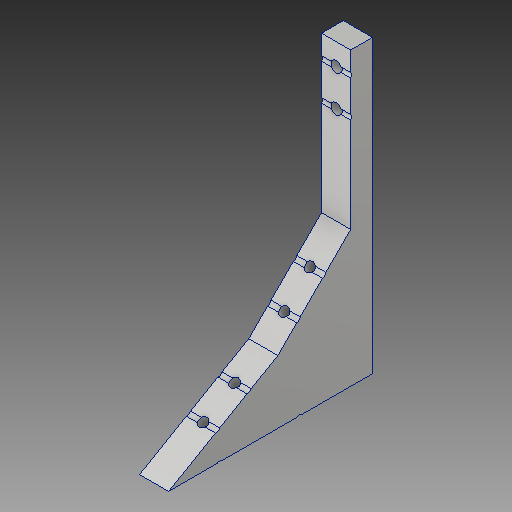
# Autodesk Inventor part: 앞판센서막이
Saved by Autodesk Inventor 2017 (Build 210142000, 142)
## iProperties
Part Number: 앞판센서막이
Material: 알루미늄 6061
Document SubType Name: Modeling
Designer: minom
Density: 2.7 g/cm^3
Appearance: 알루미늄 - 평지
Mass: 18.1843 g
Surface Area: 55.7658 cm^2
Volume: 6.73492 cm^3
Author: minom
Autodesk Inventor part; units mm, degrees
ref_plane "YZ Plane" through (0, 0, 0) normal (1, 0, 0) x (0, 1, 0)
ref_plane "XZ Plane" through (0, 0, 0) normal (0, 1, 0) x (-1, 0, 0)
sketch "스케치1" plane through (0, 0, 0) normal (1, 0, 0) x (0, 1, 0)
  line L0 (0, 0) -> (0, -30)
  line L1 (0, -30) -> (0, -50)
  line L2 (0, -50) -> (37.3205, -50)
  line L3 (0, 0) -> (17.3205, -30)
  line L4 (0, 0) -> (34.641, 0) construction
  line L5 (17.3205, -30) -> (37.3205, -50)
  line L6 (17.3205, -30) -> (43.1906, -30) construction
  line L7 (0, -30) -> (17.3205, -30)
  dimension "d0" = 30
  dimension "d1" = 20
  dimension "d2" = 60
  dimension "d3" = 45
  constraints: 16 end point, 2 horizontal, 1 collinear, 1 equal length, 1 perpendicular, 1 point on line, 1 vertical
  measures "d0" distance of L0.start L0.end
  measures "d1" distance of L0.end L1.end
  measures "d2" angle of L3 L4
  measures "d3" angle of L5 L6
extrude "돌출2" add sketch "스케치1" along normal blind 8
sketch "스케치7" plane through (8, 0, 0) normal (1, 0, 0) x (0, 0, -1)
  line L0 (50, 0) -> (50, 37.3205) projected
  line L1 (50, 0) -> (56, 0)
  line L2 (56, 0) -> (56, 80)
  line L3 (56, 80) -> (50, 80)
  line L4 (50, 80) -> (50, 0)
  point P0 (0, 0)
  dimension "d47" = 6
  dimension "d48" = 80
  constraints: 8 end point, 2 parallel, 1 horizontal, 1 perpendicular
  measures "d47" distance of L3.end L2.end
  measures "d48" distance of L2.end L1.end
extrude "돌출9" add sketch "스케치7" against normal blind 8
sketch "스케치2" plane through (0, 0, -50) normal (0, -1, 0) x (1, 0, 0)
  line L0 (0, 50) -> (0, -6) projected
  line L1 (8, 50) -> (8, -6) projected
  line L2 (0, 50) -> (8, 50) projected
  circle A0 centre (4, 36) radius 1.25
  circle A1 centre (4, 14) radius 1.25
  line L3 (8, -6) -> (0, -6) projected
  dimension "d9" = 2.5
  dimension "d10" = 2.5
  dimension "d11" = 14
  dimension "d12" = 4
  dimension "d14" = 4
  constraints: 2 centre point
  measures "d9" diameter of A0
  measures "d10" diameter of A1
  measures "d11" distance from line of L2 A0.centre
  measures "d12" distance from line of L1 A0.centre
  measures "d14" distance from line of A1.centre L1
extrude "돌출3" cut sketch "스케치2" against normal blind 4.1 contours A0 | A1
sketch "스케치3" plane through (0, 0, 0) normal (-1, 0, 0) x (0, 0, 1)
  line L0 (0, 0) -> (-56, 0) projected
  line L1 (-30, 17.3205) -> (0, 0) projected
  line L2 (-50, 37.3205) -> (-30, 17.3205) projected
  line L3 (-32.4561, 14.1197) -> (-14.9282, 4)
  line L4 (-14.9282, 4) -> (-52, 4)
  line L5 (-52, 4) -> (-52, 33.6637)
  line L6 (-52, 33.6637) -> (-32.4561, 14.1197)
  line L7 (-50, 37.3205) -> (-50, 80) projected
  line L8 (-50, 80) -> (-56, 80) projected
  line L9 (-56, 80) -> (-56, 0) projected
  dimension "d17" = 4
  dimension "d51" = 4
  dimension "d60" = 4
  constraints: 8 end point, 1 other
  measures "d17" distance between parallel lines of L2 L6
  measures "d51" distance between parallel lines of L5 L9
  measures "d60" distance between parallel lines of L1 L3
extrude "돌출4" cut sketch "스케치3" against normal blind 7 contours L3 L4 L5 L6
sketch "스케치5" plane through (0, 17.3205, -30) normal (0, 0.7071068, 0.7071068) x (1, 0, 0)
  circle A0 centre (4, 8) radius 1.6 projected
  circle A1 centre (-36, 18) radius 1.6 projected
  circle A2 centre (-255.8, 18) radius 1.6 projected
  circle A3 centre (-295.8, 18) radius 1.6 projected
  circle A4 centre (-295.8, 8) radius 1.6 projected
  circle A5 centre (-255.8, 8) radius 1.6 projected
  circle A6 centre (-36, 8) radius 1.6 projected
  circle A7 centre (4, 18) radius 1.6 projected
  line L0 (-300.9, 27) -> (9.1, 27) projected
  line L1 (-300.9, 1) -> (-300.9, 27) projected
  line L2 (9.1, 1) -> (-137.9, 1) projected
  line L3 (-153.9, 1) -> (-300.9, 1) projected
  line L4 (9.1, 27) -> (9.1, 1) projected
  circle A8 centre (4, 18) radius 1.25
  circle A9 centre (4, 8) radius 1.25
  line L5 (-153.9, 1) -> (-153.9, 8) projected
  arc A10 (-151.9, 10) -> (-153.9, 8) centre (-151.9, 8) ccw projected
  line L6 (-151.9, 10) -> (-139.9, 10) projected
  arc A11 (-137.9, 8) -> (-139.9, 10) centre (-139.9, 8) ccw projected
  line L7 (-137.9, 8) -> (-137.9, 1) projected
  circle A12 centre (-188.8, 18) radius 1.6 projected
  circle A13 centre (-103, 8) radius 1.6 projected
  circle A14 centre (-103, 18) radius 1.6 projected
  circle A15 centre (-188.8, 8) radius 1.6 projected
  point P0 (0, -33.4607)
  dimension "d24" = 2.5
  dimension "d25" = 2.5
  constraints: 2 centre point, 2 coincident
  measures "d24" diameter of A8
  measures "d25" diameter of A9
extrude "돌출6" cut sketch "스케치5" against normal blind 4.1 contours A8 | A9
sketch "스케치8" plane through (8, 37.3205, -50) normal (0, 0, 1) x (1, 0, 0)
  circle A0 centre (-303.8, 36.6795) radius 1.5 projected
  circle A1 centre (-263.8, 36.6795) radius 1.5 projected
  circle A2 centre (-44, 36.6795) radius 1.5 projected
  circle A3 centre (-4, 36.6795) radius 1.5 projected
  circle A4 centre (-4, 26.6795) radius 1.5 projected
  circle A5 centre (-44, 26.6795) radius 1.5 projected
  circle A6 centre (-263.8, 26.6795) radius 1.5 projected
  circle A7 centre (-303.8, 26.6795) radius 1.5 projected
  line L0 (-113.9, 5.6795) -> (-193.9, 5.6795) projected
  line L1 (-193.9, 5.6795) -> (-193.9, 19.6795) projected
  line L2 (-193.9, 19.6795) -> (-113.9, 19.6795) projected
  line L3 (-113.9, 19.6795) -> (-113.9, 5.6795) projected
  line L4 (-228.9, 19.6795) -> (-228.9, 5.6795) projected
  line L5 (-228.9, 5.6795) -> (-298.9, 5.6795) projected
  line L6 (-298.9, 5.6795) -> (-298.9, 19.6795) projected
  line L7 (-298.9, 19.6795) -> (-228.9, 19.6795) projected
  line L8 (-8.9, 5.6795) -> (-78.9, 5.6795) projected
  line L9 (-78.9, 5.6795) -> (-78.9, 19.6795) projected
  line L10 (-78.9, 19.6795) -> (-8.9, 19.6795) projected
  line L11 (-8.9, 19.6795) -> (-8.9, 5.6795) projected
  line L12 (1.1, 42.6795) -> (1.1, 2.6795) projected
  line L13 (-308.9, 42.6795) -> (1.1, 42.6795) projected
  line L14 (-308.9, 2.6795) -> (-308.9, 42.6795) projected
  line L15 (1.1, 2.6795) -> (-308.9, 2.6795) projected
  circle A8 centre (-4, 36.6795) radius 1.25
  circle A9 centre (-4, 26.6795) radius 1.25
  point P0 (-8, -37.3205)
  dimension "d52" = 2.5
  dimension "d53" = 2.5
  constraints: 2 centre point, 2 coincident
  measures "d52" diameter of A8
  measures "d53" diameter of A9
extrude "돌출10" cut sketch "스케치8" against normal blind 8 contours A3 | A4 | A8 | A9
ref_plane "작업 평면4" through (0, 6.4622, -11.1929) normal (0, 0.8660254, 0.5) x (1, 0, 0)
sketch "스케치9" plane through (0, 6.4622, -11.1929) normal (0, 0.8660254, 0.5) x (1, 0, 0)
  circle A0 centre (-103, 2.6003) radius 1.5 projected
  circle A1 centre (-188.8, 12.6003) radius 1.5 projected
  circle A2 centre (-188.8, 2.6003) radius 1.5 projected
  circle A3 centre (-103, 12.6003) radius 1.5 projected
  circle A4 centre (4, 12.6003) radius 1.5 projected
  circle A5 centre (-36, 2.6003) radius 1.5 projected
  circle A6 centre (-255.8, 12.6003) radius 1.5 projected
  circle A7 centre (-295.8, 12.6003) radius 1.5 projected
  circle A8 centre (-295.8, 2.6003) radius 1.5 projected
  circle A9 centre (-255.8, 2.6003) radius 1.5 projected
  circle A10 centre (-36, 12.6003) radius 1.5 projected
  circle A11 centre (4, 2.6003) radius 1.5 projected
  line L0 (-137.9, 20.6003) -> (-137.9, 13.6003) projected
  arc A12 (-139.9, 11.6003) -> (-137.9, 13.6003) centre (-139.9, 13.6003) ccw projected
  line L1 (-139.9, 11.6003) -> (-151.9, 11.6003) projected
  arc A13 (-153.9, 13.6003) -> (-151.9, 11.6003) centre (-151.9, 13.6003) ccw projected
  line L2 (-153.9, 13.6003) -> (-153.9, 20.6003) projected
  line L3 (-300.9, 20.6003) -> (-153.9, 20.6003) projected
  line L4 (-300.9, -13.3997) -> (-300.9, 20.6003) projected
  line L5 (9.1, -13.3997) -> (-300.9, -13.3997) projected
  line L6 (9.1, 20.6003) -> (9.1, -13.3997) projected
  line L7 (-137.9, 20.6003) -> (9.1, 20.6003) projected
  circle A14 centre (4, 12.6003) radius 1.25
  circle A15 centre (4, 2.6003) radius 1.25
  point P0 (0, -12.9244)
  dimension "d56" = 2.5
  dimension "d57" = 2.5
  constraints: 2 centre point, 2 coincident
  measures "d56" diameter of A14
  measures "d57" diameter of A15
extrude "돌출11" cut sketch "스케치9" against normal blind 4.1 contours A14 | A15
sketch "스케치10" plane through (8, 0, 0) normal (1, 0, 0) x (0, 0, -1)
  line L0 (14.9282, 4) -> (14.9282, 4) projected
  line L1 (12.3623, 7.1374) -> (14.5274, 8.3874) projected
  line L2 (25.1876, 9.9233) -> (23.0225, 8.6733) projected
  line L3 (21.0225, 12.1374) -> (23.1876, 13.3874) projected
  line L4 (34.773, 22.0935) -> (36.5407, 23.8612) projected
  line L5 (41.844, 29.1645) -> (43.6118, 30.9323) projected
  line L6 (56, 65.5) -> (56, 62.5) projected
  line L7 (50, 62.5) -> (50, 65.5) projected
  line L8 (56, 75.5) -> (56, 72.5) projected
  line L9 (50, 72.5) -> (50, 75.5) projected
  line L10 (14.9282, 4) -> (15.1282, 4) projected
  line L11 (15.1282, 4) -> (14.9282, 4) projected
  line L12 (15.1282, 4) -> (14.8011, 3.8111) projected
  line L13 (14.7237, 4.1) -> (14.8011, 3.8111) projected
  line L14 (14.7237, 4.1) -> (14.7237, 4.1) projected
  line L15 (14.8011, 3.8111) -> (14.7237, 4.1) projected
  line L16 (14.8011, 3.8111) -> (15.1282, 4) projected
  line L17 (14.8011, 3.8111) -> (15.1282, 4) projected
  line L18 (15.1282, 4) -> (15.1282, 4) projected
  line L19 (15.1282, 4) -> (14.8011, 3.8111) projected
  line L20 (14.8011, 3.8111) -> (14.7237, 4.1) projected
  line L21 (14.7237, 4.1) -> (14.7237, 4.1) projected
  line L22 (14.7237, 4.1) -> (14.8011, 3.8111) projected
  line L23 (15.25, 0) -> (12.75, 0) projected
  line L24 (37.25, 4) -> (34.75, 4) projected
  line L25 (37.25, 0) -> (34.75, 0) projected
  arc A0 (50, 73.3386) -> (50, 74.6614) centre (49.25, 74) ccw
  arc A1 (50, 63.3386) -> (50, 64.6614) centre (49.25, 64) ccw
  arc A2 (42.2602, 29.5807) -> (43.1956, 30.5161) centre (42.1976, 30.5788) ccw
  arc A3 (35.1891, 22.5097) -> (36.1246, 23.4451) centre (35.1265, 23.5077) ccw
  arc A4 (21.5323, 12.4317) -> (22.6779, 13.0931) centre (21.7301, 13.4119) ccw
  arc A5 (12.872, 7.4317) -> (14.0176, 8.0931) centre (13.0698, 8.4119) ccw
  arc A6 (14.6614, 0) -> (13.3386, 0) centre (14, -0.75) ccw
  arc A7 (36.6614, 0) -> (35.3386, 0) centre (36, -0.75) ccw
  dimension "d61" = 2
  dimension "d62" = 2
  dimension "d63" = 2
  dimension "d64" = 2
  dimension "d65" = 2
  dimension "d66" = 2
  dimension "d67" = 2
  dimension "d68" = 2
  dimension "d69" = 0.75
  dimension "d70" = 0.75
  dimension "d71" = 0.75
  dimension "d72" = 0.75
  dimension "d73" = 0.75
  dimension "d74" = 0.75
  dimension "d75" = 0.75
  dimension "d76" = 0.75
  constraints: 16 point on circle, 16 point on line, 8 centre point
  measures "d61" diameter of A0
  measures "d62" diameter of A1
  measures "d63" diameter of A2
  measures "d64" diameter of A3
  measures "d65" diameter of A4
  measures "d66" diameter of A5
  measures "d67" diameter of A6
  measures "d68" diameter of A7
  measures "d69" distance from line of L25 A7.centre
  measures "d70" distance from line of L23 A6.centre
  measures "d71" distance from line of L1 A5.centre
  measures "d72" distance from line of L3 A4.centre
  measures "d73" distance from line of L4 A3.centre
  measures "d74" distance from line of L5 A2.centre
  measures "d75" distance from line of L7 A1.centre
  measures "d76" distance from line of L9 A0.centre
extrude "돌출12" cut sketch "스케치10" against normal blind 8
